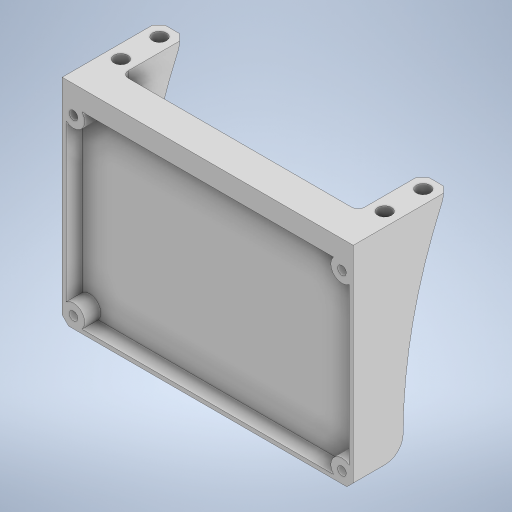
# Autodesk Inventor part: CONTROLLERMOUNT
Saved by Autodesk Inventor 2023 (Build 270158000, 158)
## iProperties
Created: 2022-08-02
Part Number: CONTROLLERMOUNT
Material: Generic
Document SubType Name: Modeling
Designer: plebbb
Density: 1 g/cm^3
Appearance: Default
Author: plebbb
Autodesk Inventor part; units mm, degrees
ref_plane "YZ Plane" through (0, 0, 0) normal (1, 0, 0) x (0, 1, 0)
ref_plane "XZ Plane" through (0, 0, 0) normal (0, 1, 0) x (-1, 0, 0)
ref_plane "XY Plane" through (0, 0, 0) normal (0, 0, 1) x (1, 0, 0)
sketch "Sketch1" plane through (0, 0, 0) normal (0, 0, 1) x (1, 0, 0)
  line L0 (0, 0) -> (90.5, 0)
  line L1 (90.5, 0) -> (90.5, 61)
  line L2 (90.5, 61) -> (0, 61)
  line L3 (0, 61) -> (0, 0)
  line L4 (3.5, 3.5) -> (87, 3.5) construction
  line L5 (87, 3.5) -> (87, 57.5) construction
  line L6 (87, 57.5) -> (3.5, 57.5) construction
  line L7 (3.5, 57.5) -> (3.5, 3.5) construction
  circle A0 centre (3.5, 57.5) radius 1.35
  circle A1 centre (3.5, 3.5) radius 1.35
  circle A2 centre (87, 3.5) radius 1.35
  circle A3 centre (87, 57.5) radius 1.35
  point P0 (3.5, 30.5)
  point P1 (0, 30.5)
  point P2 (45.25, 57.5)
  point P3 (45.25, 61)
  dimension "d0" = 54
  dimension "d1" = 83.5
  dimension "d2" = 90.5
  dimension "d3" = 61
  dimension "d4" = 2.7
  constraints: 16 end point, 4 centre point, 4 coincident, 4 midpoint, 4 parallel, 3 equal radius, 2 horizontal, 2 perpendicular, 1 horizontal alignment, 1 vertical alignment
  measures "d0" distance of L6.end L4.start
  measures "d1" distance of L5.end L6.end
  measures "d2" distance of L1.end L2.end
  measures "d3" distance of L0.end L1.end
  measures "d4" diameter of A2
extrude "Extrusion1" add sketch "Sketch1" along normal blind 5
sketch "Sketch2" plane through (0, 0, 5) normal (0, 0, 1) x (1, 0, 0)
  circle A0 centre (3.5, 3.5) radius 3.5
  circle A1 centre (3.5, 57.5) radius 3.5
  circle A2 centre (87, 57.5) radius 3.5
  circle A3 centre (87, 3.5) radius 3.5
  circle A4 centre (3.5, 3.5) radius 1.35 projected
  circle A5 centre (3.5, 57.5) radius 1.35 projected
  circle A6 centre (87, 57.5) radius 1.35 projected
  circle A7 centre (87, 3.5) radius 1.35 projected
  line L0 (1.25, 54.819) -> (1.25, 6.181)
  line L1 (6.181, 1.25) -> (84.319, 1.25)
  line L2 (89.25, 6.181) -> (89.25, 54.819)
  line L3 (84.319, 59.75) -> (6.181, 59.75)
  line L4 (3.5, 0) -> (87, 0) projected
  line L5 (3.5, 0) -> (0, 0)
  line L6 (0, 61) -> (0, 3.5) projected
  arc A8 (87, 0) -> (90.5, 3.5) centre (87, 3.5) ccw projected
  line L7 (90.5, 3.5) -> (90.5, 61) projected
  line L8 (90.5, 0) -> (90.5, 61) projected
  line L9 (90.5, 61) -> (0, 61) projected
  line L10 (0, 61) -> (0, 0) projected
  line L11 (0, 0) -> (90.5, 0) projected
  circle A9 centre (3.5, 57.5) radius 1.35 projected
  circle A10 centre (3.5, 3.5) radius 1.35 projected
  circle A11 centre (87, 3.5) radius 1.35 projected
  circle A12 centre (87, 57.5) radius 1.35 projected
  point P0 (90.5, 3.5)
  point P1 (90.5, 3.5)
  point P2 (90.5, 3.5)
  point P3 (87, 61)
  point P4 (90.5, 57.5)
  point P5 (3.5, 61)
  point P6 (0, 57.5)
  dimension "d8" = 7
  dimension "d22" = 1.25
  dimension "d23" = 1.25
  constraints: 10 end point, 8 point on circle, 4 centre point, 4 concentric, 3 equal radius, 3 perpendicular, 2 parallel, 1 horizontal, 1 vertical
  measures "d8" diameter of A2
  measures "d22" distance between parallel lines of L4 L1
  measures "d23" distance between parallel lines of L6 L0
extrude "Extrusion2" add sketch "Sketch2" along normal blind 5 contours A0 | A0 L6 A1 L0 | L1 A3 L4 A0 | A0 L5 L10 | A1 | A3 | L6 L9 A1 | A3 L8 L11 | L2 A2 L7 A3 | L9 A2 L3 A1 | A2 | L9 L7 A2
sketch "Sketch3" plane through (0, 3.5, 0) normal (-1, 0, 0) x (0, 0, 1)
  line L0 (0, 62.5) -> (-20.8334, 62.5)
  arc A0 (-7.5, 4) -> (-20.8334, 62.5) centre (-142.5, 4) ccw
  arc A1 (-7.5, 4) -> (0, -3.5) centre (0, 4) ccw
  line L1 (0, 62.5) -> (0, -3.5)
  line L2 (0, 57.5) -> (0, -3.5) projected
  arc A2 (-20, 62.5) -> (-19.2892, 59.1733) centre (-11.86, 62.5) ccw
  line L3 (0, 57.5) -> (10, 57.5) projected
  line L4 (0, 62.5) -> (10, 62.5)
  line L5 (10, -3.5) -> (10, 57.5) projected
  line L6 (10, 62.5) -> (10, 57.5)
  line L7 (0, 57.5) -> (10, 57.5) projected
  line L8 (10, 57.5) -> (0, 57.5)
  point P0 (5, 57.5)
  point P1 (5, 57.5)
  dimension "d16" = 90
  dimension "d17" = 20
  dimension "d18" = 135
  dimension "d19" = 7.5
  dimension "d27" = 5
  constraints: 10 end point, 7 point on circle, 3 centre point, 2 horizontal, 2 perpendicular, 2 point on line, 2 tangent, 1 line through centre, 1 midpoint, 1 vertical
  measures "d17" distance of L0.start A2.start
  measures "d18" radius of A0
  measures "d19" distance of L1.end A1.centre
  measures "d27" distance from line of point (5, 57.5) L0
extrude "Extrusion3" add sketch "Sketch3" against normal blind 8.5 contours L1 A1 A0 A2 L0 | L4 L6 L3 L1
sketch "Sketch4" plane through (0, 66, 0) normal (0, 1, 0) x (1, 0, 0)
  circle A0 centre (4.25, 4) radius 2.159
  circle A1 centre (4.25, 16) radius 2.159
  line L0 (0, 20) -> (8.5, 20) construction
  line L1 (4.25, 4) -> (4.25, 16) construction
  point P0 (0, 0)
  point P1 (4.25, 10)
  point P2 (4.25, 20)
  point P3 (4.25, 20)
  dimension "d28" = 4.318
  dimension "d29" = 12
  dimension "d33" = 10
  constraints: 3 midpoint, 2 centre point, 2 end point, 1 equal radius, 1 vertical, 1 vertical alignment
  measures "d28" diameter of A0
  measures "d29" distance of L1.end L1.start
  measures "d33" distance of point (4.25, 20) point (4.25, 10)
extrude "Extrusion4" cut sketch "Sketch4" against normal blind 50.25
pattern_linear "Rectangular Pattern1" count 2 spacing 82 along (1, 0, 0) of "Extrusion3", "Extrusion4"
fillet "Fillet2" radius 2 2 edges at (82, 30.5, 0) (8.5, 30.5, 0)
sketch "Sketch5" plane through (8.5, 61, 10) normal (0, 1, 0) x (1, 0, 0)
  line L0 (73.5, 0) -> (73.5, 12) projected
  arc A0 (71.5, 10) -> (73.5, 12) centre (71.5, 12) ccw projected
  line L1 (71.5, 10) -> (2, 10) projected
  arc A1 (0, 12) -> (2, 10) centre (2, 12) ccw projected
  line L2 (0, 12) -> (0, 0) projected
  line L3 (73.5, 0) -> (0, 0) projected
  point P0 (-8.5, 10)
extrude "Extrusion5" add sketch "Sketch5" along normal up to surface (5 mm away)
chamfer "Chamfer1" distance 2 angle 45 8 edges at (90.5, 0, 5) (90.5, 2.1967, -5.3033) (90.5, 35.7094, -10.4802) (90.5, 64.2991, -19.8203) (0, 0, 5) (0, 2.1967, -5.3033) (0, 35.7094, -10.4802) (0, 64.2991, -19.8203)
chamfer "Chamfer2" distance 2 angle 45 9 edges at (82, 35.7094, -10.4802) (82, 2.9585, -5.9687) (81.3185, 0.0164, -0.4961) (45.25, 0, 0) (9.1815, 0.0164, -0.4961) (8.5, 2.9585, -5.9687) (8.5, 35.7094, -10.4802) (8.5, 64.2991, -19.8203) (82, 64.2991, -19.8203)
body "Solid1"
